Autodesk Fusion 360 part; units mm, degrees
note: some values were not read from the file. Set by a fixed rule: which sketch regions a step uses.
(part 2 of 2)
  spline S140 degree 3 poles (7.5012, -18.1808) (7.4038, -17.6861) (7.3361, -17.5578) (7.1562, -17.5263) knots 0 0 0 0 1 1 1 1
  spline S141 degree 3 poles (7.1562, -17.5263) (4.7678, -17.1106) (3.7658, -16.7079) (2.6895, -15.7319) knots 0 0 0 0 1 1 1 1
  spline S142 degree 3 poles (2.6895, -15.7319) (1.4354, -14.5944) (-0.0087, -12.0031) (0.3895, -11.6049) knots 0 0 0 0 1 1 1 1
  spline S143 degree 3 poles (0.3895, -11.6049) (0.6019, -11.3927) (28.8811, -11.5856) (29.0417, -11.8004) knots 0 0 0 0 1 1 1 1
  spline S144 degree 3 poles (105.4076, -11.6917) (105.5777, -11.8967) (104.6898, -13.7091) (103.909, -14.7495) knots 0 0 0 0 1 1 1 1
  spline S145 degree 3 poles (103.909, -14.7495) (102.7287, -16.3229) (100.8745, -17.3069) (98.7533, -17.4853) knots 0 0 0 0 1 1 1 1
  spline S146 degree 3 poles (98.7533, -17.4853) (98.4015, -17.5149) (98.3888, -17.5329) (98.1583, -18.3332) knots 0 0 0 0 1 1 1 1
  spline S147 degree 3 poles (98.1583, -18.3332) (97.4016, -20.9629) (95.7905, -22.2874) (93.0865, -22.5031) knots 0 0 0 0 1 1 1 1
  spline S148 degree 3 poles (93.0865, -22.5031) (91.9853, -22.5909) (91.9718, -22.5999) (91.512, -23.5302) knots 0 0 0 0 1 1 1 1
  spline S149 degree 3 poles (91.512, -23.5302) (90.083, -26.4216) (88.5933, -26.9034) (81.1207, -26.8909) knots 0 0 0 0 1 1 1 1
  line L26 (81.1207, -26.8909) -> (76.4524, -26.883)
  line L27 (76.4524, -26.883) -> (75.4002, -27.5833)
  spline S150 degree 3 poles (75.4002, -27.5833) (72.2596, -29.6741) (69.9151, -30.3178) (65.4579, -30.313) knots 0 0 0 0 1 1 1 1
  spline S151 degree 3 poles (65.4579, -30.313) (62.0784, -30.3096) (60.5256, -30.071) (61.4124, -29.6913) knots 0 0 0 0 1 1 1 1
  spline S152 degree 3 poles (61.4124, -29.6913) (69.2838, -26.3223) (73.3494, -21.73) (76.2508, -12.9305) knots 0 0 0 0 1 1 1 1
  spline S153 degree 3 poles (76.2508, -12.9305) (76.5514, -12.0187) (76.7001, -11.7105) (76.8728, -11.6409) knots 0 0 0 0 1 1 1 1
  spline S154 degree 3 poles (76.8728, -11.6409) (77.3118, -11.4636) (105.2597, -11.5133) (105.4076, -11.6917) knots 0 0 0 0 1 1 1 1
  spline S155 degree 3 poles (53.5757, -28.2575) (53.7787, -28.6359) (54.2909, -29.6122) (54.7142, -30.4271) knots 0 0 0 0 1 1 1 1
  spline S156 degree 3 poles (54.7142, -30.4271) (55.1378, -31.242) (55.5908, -32.0992) (55.7213, -32.3321) knots 0 0 0 0 1 1 1 1
  spline S157 degree 3 poles (55.7213, -32.3321) (55.9797, -32.794) (56.5094, -33.786) (57.3315, -35.3483) knots 0 0 0 0 1 1 1 1
  spline S158 degree 3 poles (57.3315, -35.3483) (57.6225, -35.9013) (58.1803, -36.9604) (58.5711, -37.7021) knots 0 0 0 0 1 1 1 1
  spline S159 degree 3 poles (58.5711, -37.7021) (59.3881, -39.2528) (59.3881, -39.3023) (58.5674, -39.7404) knots 0 0 0 0 1 1 1 1
  spline S160 degree 3 poles (58.5674, -39.7404) (57.4249, -40.3505) (56.5007, -41.7282) (56.0737, -43.4578) knots 0 0 0 0 1 1 1 1
  spline S161 degree 3 poles (56.0737, -43.4578) (55.8157, -44.5034) (55.6953, -52.0335) (55.9329, -52.2698) knots 0 0 0 0 1 1 1 1
  spline S162 degree 3 poles (55.9329, -52.2698) (55.9911, -52.3274) (56.624, -52.4957) (57.3394, -52.6436) knots 0 0 0 0 1 1 1 1
  spline S163 degree 3 poles (57.3394, -52.6436) (68.5721, -54.9661) (76.9207, -64.6679) (77.4586, -76.0235) knots 0 0 0 0 1 1 1 1
  spline S164 degree 3 poles (77.4586, -76.0235) (77.5457, -77.8626) (76.9906, -77.6817) (82.5437, -77.6814) knots 0 0 0 0 1 1 1 1
  spline S165 degree 3 poles (82.5437, -77.6814) (89.9986, -77.6809) (91.7713, -77.185) (92.9434, -74.7731) knots 0 0 0 0 1 1 1 1
  spline S166 degree 3 poles (92.9434, -74.7731) (93.2545, -74.1323) (93.2386, -74.1288) (95.5926, -75.3689) knots 0 0 0 0 1 1 1 1
  spline S167 degree 3 poles (95.5926, -75.3689) (96.7139, -75.9595) (97.9646, -76.6061) (98.3721, -76.8059) knots 0 0 0 0 1 1 1 1
  spline S168 degree 3 poles (98.3721, -76.8059) (99.3873, -77.3033) (99.9744, -77.6097) (103.1346, -79.2906) knots 0 0 0 0 1 1 1 1
  spline S169 degree 3 poles (103.1346, -79.2906) (103.6585, -79.5695) (104.3355, -79.9259) (104.6393, -80.0828) knots 0 0 0 0 1 1 1 1
  spline S170 degree 3 poles (104.6393, -80.0828) (105.7077, -80.6349) (105.745, -80.5974) (102.3938, -82.3381) knots 0 0 0 0 1 1 1 1
  spline S171 degree 3 poles (102.3938, -82.3381) (101.5788, -82.7611) (100.2691, -83.4538) (99.4833, -83.8771) knots 0 0 0 0 1 1 1 1
  spline S172 degree 3 poles (99.4833, -83.8771) (92.9315, -87.4064) (93.3381, -87.2543) (92.8299, -86.3661) knots 0 0 0 0 1 1 1 1
  spline S173 degree 3 poles (92.8299, -86.3661) (92.189, -85.2466) (91.1524, -84.4748) (89.5879, -83.9528) knots 0 0 0 0 1 1 1 1
  line L28 (89.5879, -83.9528) -> (88.7412, -83.6702)
  line L29 (88.7412, -83.6702) -> (82.9747, -83.6343)
  spline S174 degree 3 poles (82.9747, -83.6343) (79.8028, -83.6144) (77.1062, -83.6237) (76.9818, -83.6546) knots 0 0 0 0 1 1 1 1
  spline S175 degree 3 poles (76.9818, -83.6546) (76.7334, -83.7171) (76.6884, -83.8144) (76.1971, -85.3546) knots 0 0 0 0 1 1 1 1
  spline S176 degree 3 poles (76.1971, -85.3546) (74.9771, -89.1794) (72.5048, -93.1447) (69.433, -96.2041) knots 0 0 0 0 1 1 1 1
  spline S177 degree 3 poles (69.433, -96.2041) (67.3505, -98.2782) (67.3627, -98.2694) (58.4017, -104.2167) knots 0 0 0 0 1 1 1 1
  spline S178 degree 3 poles (58.4017, -104.2167) (57.1402, -105.0539) (56.0448, -105.8151) (55.9676, -105.9082) knots 0 0 0 0 1 1 1 1
  spline S179 degree 3 poles (55.9676, -105.9082) (55.8522, -106.0471) (55.8271, -108.7729) (55.8271, -121.1159) knots 0 0 0 0 1 1 1 1
  line L30 (55.8271, -121.1159) -> (55.8271, -136.1546)
  line L31 (55.8271, -136.1546) -> (56.5968, -137.2021)
  spline S180 degree 3 poles (56.5968, -137.2021) (61.9141, -144.4395) (62.1768, -152.2381) (57.3225, -158.7447) knots 0 0 0 0 1 1 1 1
  spline S181 degree 3 poles (57.3225, -158.7447) (56.1684, -160.2917) (56.1975, -160.1888) (56.6502, -161.1037) knots 0 0 0 0 1 1 1 1
  spline S182 degree 3 poles (56.6502, -161.1037) (57.1582, -162.1306) (57.6546, -162.6846) (58.5343, -163.2074) knots 0 0 0 0 1 1 1 1
  spline S183 degree 3 poles (58.5343, -163.2074) (59.4135, -163.7297) (59.4098, -163.6879) (58.6962, -165.0315) knots 0 0 0 0 1 1 1 1
  spline S184 degree 3 poles (58.6962, -165.0315) (57.7532, -166.806) (55.2585, -171.5315) (54.6367, -172.72) knots 0 0 0 0 1 1 1 1
  spline S185 degree 3 poles (54.6367, -172.72) (52.6619, -176.4948) (53.0103, -176.4133) (51.463, -173.4608) knots 0 0 0 0 1 1 1 1
  spline S186 degree 3 poles (51.463, -173.4608) (49.9213, -170.5192) (49.5795, -169.8699) (49.3178, -169.3863) knots 0 0 0 0 1 1 1 1
  spline S187 degree 3 poles (49.3178, -169.3863) (49.1604, -169.0952) (48.7079, -168.238) (48.3127, -167.4813) knots 0 0 0 0 1 1 1 1
  spline S188 degree 3 poles (48.3127, -167.4813) (47.9171, -166.7245) (47.3387, -165.6406) (47.0273, -165.0725) knots 0 0 0 0 1 1 1 1
  spline S189 degree 3 poles (47.0273, -165.0725) (46.314, -163.7715) (46.3145, -163.7176) (47.0469, -163.2984) knots 0 0 0 0 1 1 1 1
  spline S190 degree 3 poles (47.0469, -163.2984) (47.8713, -162.827) (48.5891, -162.0554) (49.0379, -161.1585) knots 0 0 0 0 1 1 1 1
  spline S191 degree 3 poles (49.0379, -161.1585) (49.824, -159.5882) (49.7861, -160.0983) (49.8221, -150.5365) knots 0 0 0 0 1 1 1 1
  line L32 (49.8221, -150.5365) -> (49.8546, -141.9529)
  line L33 (49.8546, -141.9529) -> (49.2424, -141.3753)
  spline S192 degree 3 poles (49.2424, -141.3753) (48.9058, -141.0576) (48.3013, -140.4914) (47.8991, -140.1167) knots 0 0 0 0 1 1 1 1
  spline S193 degree 3 poles (47.8991, -140.1167) (46.708, -139.0068) (46.6587, -138.9565) (45.4086, -137.5807) knots 0 0 0 0 1 1 1 1
  spline S194 degree 3 poles (45.4086, -137.5807) (36.6586, -127.9506) (34.8462, -118.4587) (39.9915, -109.2092) knots 0 0 0 0 1 1 1 1
  spline S195 degree 3 poles (39.9915, -109.2092) (41.8846, -105.8058) (45.3491, -102.0646) (48.8032, -99.6926) knots 0 0 0 0 1 1 1 1
  spline S196 degree 3 poles (48.8032, -99.6926) (49.3059, -99.3476) (49.7464, -98.9888) (49.7821, -98.8952) knots 0 0 0 0 1 1 1 1
  spline S197 degree 3 poles (49.7821, -98.8952) (49.9155, -98.5478) (49.8557, -83.8705) (49.7205, -83.7353) knots 0 0 0 0 1 1 1 1
  spline S198 degree 3 poles (49.7205, -83.7353) (49.5059, -83.5208) (37.2671, -83.5552) (37.1843, -83.7708) knots 0 0 0 0 1 1 1 1
  spline S199 degree 3 poles (37.1843, -83.7708) (36.93, -84.4338) (38.1947, -86.115) (39.583, -86.959) knots 0 0 0 0 1 1 1 1
  spline S200 degree 3 poles (39.583, -86.959) (41.542, -88.1502) (42.3945, -89.4223) (42.3741, -91.123) knots 0 0 0 0 1 1 1 1
  spline S201 degree 3 poles (42.3741, -91.123) (42.3423, -93.7702) (41.5531, -97.3757) (40.5252, -99.5691) knots 0 0 0 0 1 1 1 1
  spline S202 degree 3 poles (40.5252, -99.5691) (39.0938, -102.6234) (37.7978, -103.0981) (34.8464, -101.6487) knots 0 0 0 0 1 1 1 1
  spline S203 degree 3 poles (34.8464, -101.6487) (32.3424, -100.4189) (28.2337, -96.8153) (27.4521, -95.1627) knots 0 0 0 0 1 1 1 1
  spline S204 degree 3 poles (27.4521, -95.1627) (26.9311, -94.0615) (27.1865, -91.4784) (28.0133, -89.4821) knots 0 0 0 0 1 1 1 1
  spline S205 degree 3 poles (28.0133, -89.4821) (28.7433, -87.72) (28.8041, -87.109) (28.4035, -85.5662) knots 0 0 0 0 1 1 1 1
  spline S206 degree 3 poles (28.4035, -85.5662) (28.2525, -84.9842) (28.1054, -84.3799) (28.0763, -84.2232) knots 0 0 0 0 1 1 1 1
  spline S207 degree 3 poles (28.0763, -84.2232) (27.9556, -83.57) (28.1699, -83.5919) (22.3155, -83.6359) knots 0 0 0 0 1 1 1 1
  spline S208 degree 3 poles (22.3155, -83.6359) (16.4042, -83.6806) (16.4767, -83.6729) (14.9963, -84.4182) knots 0 0 0 0 1 1 1 1
  spline S209 degree 3 poles (14.9963, -84.4182) (14.1057, -84.8667) (13.3088, -85.589) (12.8929, -86.3248) knots 0 0 0 0 1 1 1 1
  spline S210 degree 3 poles (12.8929, -86.3248) (12.4172, -87.1667) (12.4336, -87.1635) (11.367, -86.6114) knots 0 0 0 0 1 1 1 1
  spline S211 degree 3 poles (11.367, -86.6114) (10.0155, -85.9115) (7.094, -84.3571) (6.7204, -84.1391) knots 0 0 0 0 1 1 1 1
  spline S212 degree 3 poles (6.7204, -84.1391) (6.5458, -84.0372) (5.5597, -83.5173) (4.5291, -82.9839) knots 0 0 0 0 1 1 1 1
  spline S213 degree 3 poles (4.5291, -82.9839) (0.317, -80.8035) (0.0415, -80.5998) (0.7938, -80.2203) knots 0 0 0 0 1 1 1 1
  spline S214 degree 3 poles (0.7938, -80.2203) (0.9684, -80.1322) (2.3236, -79.4179) (3.8055, -78.6328) knots 0 0 0 0 1 1 1 1
  spline S215 degree 3 poles (3.8055, -78.6328) (5.2874, -77.8478) (6.6225, -77.1578) (6.7723, -77.0996) knots 0 0 0 0 1 1 1 1
  spline S216 degree 3 poles (6.7723, -77.0996) (7.0197, -77.0035) (8.8527, -76.0529) (11.389, -74.7054) knots 0 0 0 0 1 1 1 1
  spline S217 degree 3 poles (11.389, -74.7054) (12.4833, -74.1238) (12.4047, -74.1053) (12.9593, -75.0761) knots 0 0 0 0 1 1 1 1
  spline S218 degree 3 poles (12.9593, -75.0761) (14.1848, -77.2218) (15.8591, -77.6732) (22.6142, -77.6785) knots 0 0 0 0 1 1 1 1
  spline S219 degree 3 poles (22.6142, -77.6785) (27.5323, -77.6822) (27.0433, -77.8558) (27.1399, -76.0722) knots 0 0 0 0 1 1 1 1
  spline S220 degree 3 poles (27.1399, -76.0722) (27.2928, -73.2531) (27.8384, -70.838) (28.9997, -67.8392) knots 0 0 0 0 1 1 1 1
  spline S221 degree 3 poles (28.9997, -67.8392) (32.1093, -59.8101) (40.0465, -53.6027) (48.7519, -52.392) knots 0 0 0 0 1 1 1 1
  spline S222 degree 3 poles (48.7519, -52.392) (49.1987, -52.3298) (49.6311, -52.2237) (49.7126, -52.156) knots 0 0 0 0 1 1 1 1
  spline S223 degree 3 poles (49.7126, -52.156) (49.9496, -51.9594) (49.8528, -44.1156) (49.6025, -43.2329) knots 0 0 0 0 1 1 1 1
  spline S224 degree 3 poles (49.6025, -43.2329) (49.1487, -41.6332) (48.1534, -40.2537) (47.0408, -39.6814) knots 0 0 0 0 1 1 1 1
  spline S225 degree 3 poles (47.0408, -39.6814) (46.2219, -39.2605) (45.979, -39.8325) (50.9035, -30.5858) knots 0 0 0 0 1 1 1 1
  spline S226 degree 3 poles (50.9035, -30.5858) (52.9915, -26.665) (52.8082, -26.8248) (53.5757, -28.2575) knots 0 0 0 0 1 1 1 1
  spline S227 degree 3 poles (48.8421, -63.0425) (43.7158, -64.1869) (39.0718, -68.2715) (37.2637, -73.2258) knots 0 0 0 0 1 1 1 1
  spline S228 degree 3 poles (37.2637, -73.2258) (36.6496, -74.9086) (36.2474, -77.2036) (36.5109, -77.5211) knots 0 0 0 0 1 1 1 1
  spline S229 degree 3 poles (36.5109, -77.5211) (36.7361, -77.7923) (49.4258, -77.7605) (49.6723, -77.4883) knots 0 0 0 0 1 1 1 1
  spline S230 degree 3 poles (49.6723, -77.4883) (49.9345, -77.1983) (49.9422, -63.1357) (49.68, -63.0351) knots 0 0 0 0 1 1 1 1
  spline S231 degree 3 poles (49.68, -63.0351) (49.4983, -62.9653) (49.1757, -62.9682) (48.8421, -63.0425) knots 0 0 0 0 1 1 1 1
  spline S232 degree 3 poles (55.8808, -63.3928) (55.6453, -63.8323) (55.7906, -77.3546) (56.0324, -77.5314) knots 0 0 0 0 1 1 1 1
  spline S233 degree 3 poles (56.0324, -77.5314) (56.3356, -77.7531) (67.8035, -77.7555) (68.1064, -77.534) knots 0 0 0 0 1 1 1 1
  spline S234 degree 3 poles (68.1064, -77.534) (68.2969, -77.3949) (68.3006, -77.3345) (68.1733, -76.4492) knots 0 0 0 0 1 1 1 1
  spline S235 degree 3 poles (68.1733, -76.4492) (67.3222, -70.5326) (63.0415, -65.3928) (57.3945, -63.5074) knots 0 0 0 0 1 1 1 1
  spline S236 degree 3 poles (57.3945, -63.5074) (56.2533, -63.1264) (56.0324, -63.1095) (55.8808, -63.3928) knots 0 0 0 0 1 1 1 1
  spline S237 degree 3 poles (55.8774, -83.8798) (55.7295, -84.2687) (55.7398, -94.9079) (55.8885, -95.3341) knots 0 0 0 0 1 1 1 1
  spline S238 degree 3 poles (55.8885, -95.3341) (56.029, -95.7379) (56.0615, -95.7281) (57.7929, -94.769) knots 0 0 0 0 1 1 1 1
  spline S239 degree 3 poles (57.7929, -94.769) (62.4517, -92.1874) (65.8707, -88.4806) (67.2645, -84.4997) knots 0 0 0 0 1 1 1 1
  spline S240 degree 3 poles (67.2645, -84.4997) (67.6026, -83.5337) (68.0728, -83.6083) (61.6487, -83.6083) knots 0 0 0 0 1 1 1 1
  line L34 (61.6487, -83.6083) -> (55.9805, -83.6083)
  line L35 (55.9805, -83.6083) -> (55.8774, -83.8798)
  spline S241 degree 3 poles (49.0731, -113.0035) (46.0812, -117.9714) (46.101, -123.5628) (49.1273, -128.3465) knots 0 0 0 0 1 1 1 1
  spline S242 degree 3 poles (49.1273, -128.3465) (49.8811, -129.5381) (49.8475, -129.8977) (49.8475, -120.65) knots 0 0 0 0 1 1 1 1
  spline S243 degree 3 poles (49.8475, -120.65) (49.8475, -111.3129) (49.8827, -111.6592) (49.0731, -113.0035) knots 0 0 0 0 1 1 1 1
extrude "Extrude1" [suppressed]
extrude "Extrude2" [suppressed]
